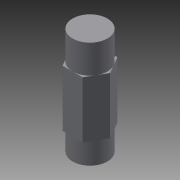
# Autodesk Inventor part: Elevator Gearbox Hex
Saved by Autodesk Inventor 2015 (Build 190159000, 159)
## iProperties
Created: 2015-02-17
Part Number: Elevator Gearbox Hex
Material: Generic
Document SubType Name: Modeling
Designer: chapale16
Density: 1 g/cm^3
Appearance: Default
Author: chapale16
Autodesk Inventor part; units mm, degrees
ref_plane "YZ Plane" through (0, 0, 0) normal (1, 0, 0) x (0, 1, 0)
ref_plane "XZ Plane" through (0, 0, 0) normal (0, 1, 0) x (-1, 0, 0)
ref_plane "XY Plane" through (0, 0, 0) normal (0, 0, 1) x (1, 0, 0)
sketch "Sketch1" plane through (0, 0, 0) normal (0, 1, 0) x (-1, 0, 0)
  line L0 (-3.6631, -6.3447) -> (-7.3262, 0)
  line L1 (-7.3262, 0) -> (-3.6631, 6.3447)
  line L2 (-3.6631, 6.3447) -> (3.6631, 6.3447)
  line L3 (3.6631, 6.3447) -> (7.3262, 0)
  line L4 (7.3262, 0) -> (3.6631, -6.3447)
  line L5 (3.6631, -6.3447) -> (-3.6631, -6.3447)
  point P0 (0, 0)
  point P1 (0, 0)
  constraints: 12 end point, 1 coincident, 13 other
extrude "Extrusion1" add sketch "Sketch1" along normal blind 38.862
sketch "Sketch2" plane through (0, 38.862, 0) normal (0, 1, 0) x (1, 0, 0)
  circle A0 centre (0, 0) radius 6.3447
  line L0 (-3.6631, 6.3447) -> (-7.3262, 0) projected
  line L1 (-12.7498, -15.4851) -> (22.5218, -15.4851)
  line L2 (22.5218, -15.4851) -> (22.5218, 21.9986)
  line L3 (22.5218, 21.9986) -> (-12.7498, 21.9986)
  line L4 (-12.7498, 21.9986) -> (-12.7498, -15.4851)
  constraints: 8 end point, 2 parallel, 1 centre point, 1 coincident, 1 horizontal, 1 perpendicular, 1 tangent
extrude "Extrusion2" cut sketch "Sketch2" against normal blind 10.414
sketch "Sketch3" plane through (0, 0, 0) normal (0, -1, 0) x (1, 0, 0)
  circle A0 centre (0, 0) radius 6.3447
  line L0 (13.1193, 9.9547) -> (-18.5882, 9.9547)
  line L1 (-18.5882, 9.9547) -> (-18.5882, -22.736)
  line L2 (-18.5882, -22.736) -> (13.1193, -22.736)
  line L3 (13.1193, -22.736) -> (13.1193, 9.9547)
  constraints: 8 end point, 2 parallel, 1 centre point, 1 coincident, 1 horizontal, 1 perpendicular
extrude "Extrusion3" cut sketch "Sketch3" against normal blind 7.874
body "Solid1"
